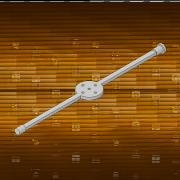
# Autodesk Inventor part: MotorMount_Part
Saved by Autodesk Inventor 2017 (Build 210142000, 142)
## iProperties
Created: 2017-01-13
Part Number: MotorMount_Part
Material: Generic
Document SubType Name: Modeling
Designer: David Kopala
Density: 1 g/cm^3
Appearance: Default
Author: David Kopala
Autodesk Inventor part; units mm, degrees
ref_plane "YZ Plane" through (0, 0, 0) normal (1, 0, 0) x (0, 1, 0)
ref_plane "XZ Plane" through (0, 0, 0) normal (0, 1, 0) x (-1, 0, 0)
ref_plane "XY Plane" through (0, 0, 0) normal (0, 0, 1) x (1, 0, 0)
sketch "Sketch1" plane through (0, 0, 0) normal (0, 0, 1) x (1, 0, 0)
  line L0 (0, 0) -> (7.62, 0)
  line L1 (7.62, 0) -> (7.62, 5.08)
  line L2 (7.62, 5.08) -> (0, 5.08)
  line L3 (0, 5.08) -> (0, 0)
  dimension "d0" = 7.62
  dimension "d1" = 5.08
  constraints: 8 end point, 2 parallel, 1 horizontal, 1 perpendicular
  measures "d0" distance of L2.end L1.end
  measures "d1" distance of L1.end L0.end
extrude "Extrusion1" add sketch "Sketch1" along normal blind 259.8166
sketch "Sketch2" plane through (0, 0, 259.8166) normal (0, 0, 1) x (1, 0, 0)
  circle A0 centre (3.8115, 2.54) radius 5.08
  line L0 (7.62, 5.08) -> (0, 5.08) projected
  line L1 (7.62, 0) -> (7.62, 5.08) projected
  point P0 (0, 0)
  dimension "d4" = 10.16
  dimension "d5" = 2.54
  dimension "d6" = 3.8085
  constraints: 1 centre point
  measures "d4" diameter of A0
  measures "d5" distance from line of A0.centre L0
  measures "d6" distance from line of L1 A0.centre
extrude "Extrusion2" add sketch "Sketch2" along normal blind 12.7
sketch "Sketch3" plane through (0, 0, 0) normal (0, 0, -1) x (-1, 0, 0)
  circle A0 centre (-3.8115, 2.54) radius 5.08
  circle A1 centre (-3.8115, 2.54) radius 5.08 projected
  point P0 (0, 0)
  dimension "d9" = 10.16
  constraints: 1 centre point, 1 concentric
  measures "d9" diameter of A0
extrude "Extrusion3" add sketch "Sketch3" along normal blind 12.7
sketch "Sketch4" plane through (3.8115, 2.54, -12.7) normal (0, 0, -1) x (-1, 0, 0)
  circle A0 centre (0, 0) radius 7.62
  point P0 (3.8115, -2.54)
  dimension "d12" = 15.24
  constraints: 1 centre point
  measures "d12" diameter of A0
extrude "Extrusion4" add sketch "Sketch4" along normal blind 3.175
sketch "Sketch5" plane through (0, 5.08, 259.8166) normal (0, 1, 0) x (1, 0, 0)
  line L0 (7.62, 259.8166) -> (7.62, 0) projected
  line L1 (-1.2685, 259.8166) -> (8.8915, 259.8166) projected
  circle A0 centre (4.445, 129.9083) radius 20
  point P0 (0, 259.8166)
  dimension "d15" = 3.175
  dimension "d16" = 259.8166
  dimension "d17" = 129.9083
  dimension "d18" = 40
  constraints: 1 centre point, 1 coincident
  measures "d15" distance from line of L0 point (4.445, 129.908)
  measures "d16" distance of L0.start L0.end
  measures "d17" distance from line of L1 point (4.445, 129.908)
  measures "d18" diameter of A0
extrude "Extrusion5" add sketch "Sketch5" against normal up to surface (5.08 mm away)
sketch "Sketch6" plane through (0, 5.08, 259.8166) normal (0, 1, 0) x (1, 0, 0)
  circle A0 centre (4.445, 129.9083) radius 20
  arc A1 (0, 149.4081) -> (0, 110.4085) centre (4.445, 129.9083) ccw projected
  circle A2 centre (4.445, 129.9083) radius 12.5
  point P0 (0, 259.8166)
  point P1 (-8.055, 129.9083)
  point P2 (4.445, 142.4083)
  point P3 (16.945, 129.9083)
  point P4 (4.445, 117.4083)
  dimension "d21" = 40
  dimension "d22" = 0
  dimension "d23" = 0
  dimension "d24" = 25
  constraints: 4 point on circle, 2 centre point, 2 coincident
  measures "d21" diameter of A0
  measures "d22" distance of A1.centre A0.centre
  measures "d23" distance of A1.centre A0.centre
  measures "d24" diameter of A2
hole "Hole1" at (4.445, 5.08, 129.9083) at (-8.055, 5.08, 129.9083) at (4.445, 5.08, 117.4083) at (16.945, 5.08, 129.9083) at (4.445, 5.08, 142.4083) direction (0, -1, 0) diameter 4 end through all
body "Solid1"
